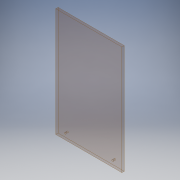
# Autodesk Inventor part: EBF_005.1-bottom-plate_cup-holder
Saved by Autodesk Inventor 2019 (Build 230136000, 136)
## iProperties
Created: 2019-02-28
Part Number: EBF_005.1-bottom-plate_cup-holder
Material: Generic
Document SubType Name: Modeling
Designer: Rene
Density: 1 g/cm^3
Appearance: Polycarbonate - Smoked
Author: Rene
Autodesk Inventor part; units mm, degrees
ref_plane "YZ Plane" through (0, 0, 0) normal (1, 0, 0) x (0, 1, 0)
ref_plane "XZ Plane" through (0, 0, 0) normal (0, 1, 0) x (-1, 0, 0)
ref_plane "XY Plane" through (0, 0, 0) normal (0, 0, 1) x (1, 0, 0)
sketch "Sketch1" plane through (0, 0, 0) normal (0, 0, 1) x (1, 0, 0)
  line L0 (-70, -115) -> (70, -115)
  line L1 (70, -115) -> (70, 115)
  line L2 (70, 115) -> (-70, 115)
  line L3 (-70, 115) -> (-70, -115)
  point P0 (0, 0)
  dimension "width" = 140
  dimension "d1" = 70
  dimension "d2" = 230
  dimension "d3" = 115
  constraints: 8 end point, 2 parallel, 1 horizontal, 1 perpendicular
  measures "width" distance of L0.start L0.end
  measures "d1" horizontal distance of point (0, 0) L0.start
  measures "d2" distance of L2.end L0.start
  measures "d3" vertical distance of point (0, 0) L0.start
extrude "Extrusion1" add sketch "Sketch1" along normal blind 5
sketch "Sketch3" plane through (0, 0, 5) normal (0, 0, 1) x (1, 0, 0)
  line L0 (-70, 115) -> (-70, -115) projected
  line L1 (-70, -115) -> (70, -115) projected
  point P0 (0, 0)
  point P1 (-50, -103)
  point P2 (50, -103)
  dimension "d33" = 20
  dimension "d34" = 12
  dimension "d35" = 12
  dimension "d36" = 20
  measures "d33" distance from line of point (-50, -103) L0
  measures "d34" distance from line of L1 point (50, -103)
  measures "d35" vertical distance of L0.end point (-50, -103)
  measures "d36" horizontal distance of L1.end point (50, -103)
hole "Hole1" at (-50, -103, 5) at (50, -103, 5) direction (0, 0, -1) diameter 3.5 end through all
equation "\"d1\" = 0.5 * width"
equation "\"d3\" = 0.5 * d2"
equation "\"d35\" = d34"
equation "\"d36\" = d33"
body "Solid1"
